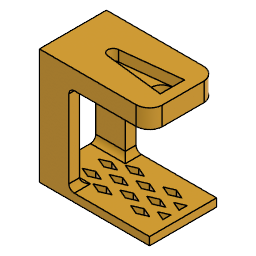
femur (Autodesk Fusion 360 design; units mm, degrees)
part number: 2026-05-23-05-17-23-124
Autodesk Fusion 360 part; units mm, degrees
note: some values were not read from the file. Set by a fixed rule: which face or edge a step refers to.
sketch "Sketch1" plane through (0, 0, 0) normal (0, 1, 0) x (1, 0, 0)
  line L0 (0, 0) -> (0, -33)
  line L1 (0, -33) -> (41, -33)
  line L2 (41, -33) -> (41, 0)
  line L3 (41, 0) -> (0, 0)
  dimension "d1" = 33
  dimension "d2" = 41
  constraint coincident L0.start L3.end
  constraint vertical L0
  constraint perpendicular L0 L1
  constraint perpendicular L1 L2
  constraint perpendicular L0 L3
  measures "d1" distance of L0.start L0.end
  measures "d2" distance of L0.end L1.end
extrude "Extrude1" add sketch "Sketch1" along normal blind 3 contours L0 L1 L2 L3 picked at (13.666667, -22)
sketch "Sketch2" plane through (0, 3, 0) normal (0, 1, 0) x (-1, 0, 0)
  line L0 (-41, 0) -> (0, 0)
  line L1 (0, 0) -> (0, 33)
  line L2 (0, 33) -> (-41, 33)
  line L3 (-41, 33) -> (-41, 0)
  line L4 (-41, 33) -> (-41, 30)
  line L5 (-41, 30) -> (0, 30)
  line L6 (0, 30) -> (0, 33)
  line L7 (0, 33) -> (-41, 33)
  line L8 (-41, 0) -> (-41, 3)
  line L9 (-41, 3) -> (0, 3)
  line L10 (0, 3) -> (0, 0)
  line L11 (0, 0) -> (-41, 0)
  constraint coincident L2.end L3.start
  constraint coincident L3 L4.end
  constraint coincident L1 L5.end
  constraint perpendicular L1 L5
  constraint coincident L1.end L2.start
  constraint coincident L0.start L3.end
  constraint coincident L3 L8.end
  constraint coincident L1 L9.end
  constraint perpendicular L1 L9
  constraint coincident L0.end L1.start
extrude "Extrude2" add sketch "Sketch2" along normal blind 15 contours L0 L1 L3 L8 L9 L10 L11 | L1 L2 L3 L4 L5 L6 L7 picked at (-27.333333, 2) picked at (-27.333333, 32)
sketch "Sketch3" plane through (0, 18, 0) normal (0, 1, 0) x (-1, 0, 0)
  line L0 (0, 33) -> (-41, 33)
  line L1 (-41, 33) -> (-41, 30)
  line L2 (-41, 30) -> (0, 30)
  line L3 (0, 30) -> (0, 33)
  line L4 (-41, 33) -> (-41, 30)
  line L5 (-41, 30) -> (0, 30)
  line L6 (0, 30) -> (0, 33)
  line L7 (0, 33) -> (-41, 33)
  line L8 (-41, 30) -> (-38.000001, 30)
  line L9 (-38.000001, 30) -> (-38.000001, 0)
  line L10 (-38.000001, 0) -> (-41, 0)
  line L11 (-41, 0) -> (-41, 30)
  line L12 (0, 0) -> (-3, 0)
  line L13 (-3, 0) -> (-3, 30)
  line L14 (0, 30) -> (0, 0)
  line L15 (-41.000001, 3) -> (0, 3)
  line L16 (0, 0) -> (-38.000001, 0)
  line L17 (-38.000001, 30) -> (-31.000001, 30)
  line L18 (-31.000001, 30) -> (-24.000001, 30)
  line L19 (-24.000001, 30) -> (-17.000001, 30)
  line L20 (-17.000001, 30) -> (-10.000001, 30)
  line L21 (-10.000001, 30) -> (-3, 30)
  line L22 (-38.000001, 30) -> (-38.000001, 24.6)
  line L23 (-38.000001, 24.6) -> (-38.000001, 19.2)
  line L24 (-38.000001, 19.2) -> (-38.000001, 13.8)
  line L25 (-38.000001, 13.8) -> (-38.000001, 8.4)
  line L26 (-38.000001, 3) -> (-31.000001, 3)
  line L27 (-31.000001, 3) -> (-24.000001, 3)
  line L28 (-24.000001, 3) -> (-17.000001, 3)
  line L29 (-17.000001, 3) -> (-10, 3)
  line L30 (-3, 3) -> (-3, 8.4)
  line L31 (-3, 8.4) -> (-3, 13.8)
  line L32 (-3, 13.8) -> (-3, 19.2)
  line L33 (-3, 19.2) -> (-3, 24.6)
  line L34 (-38.000001, 30) -> (-3, 3)
  line L35 (-38.000001, 24.6) -> (-10, 3)
  line L36 (-38.000001, 19.2) -> (-17.000001, 3)
  line L37 (-38.000001, 13.8) -> (-24, 3)
  line L38 (-38.000001, 8.4) -> (-31.000001, 3)
  line L39 (-31.000001, 30) -> (-3, 8.4)
  line L40 (-24.000001, 30) -> (-3, 13.8)
  line L41 (-17.000001, 30) -> (-3, 19.2)
  line L42 (-10.000001, 30) -> (-3, 24.6)
  line L43 (-3, 30) -> (-38.000001, 3)
  line L44 (-3, 24.6) -> (-31.000001, 3)
  line L45 (-3, 19.2) -> (-24.000001, 3)
  line L46 (-3, 13.8) -> (-17.000001, 3)
  line L47 (-3, 8.4) -> (-10, 3)
  line L48 (-10.000001, 30) -> (-38.000001, 8.4)
  line L49 (-17.000001, 30) -> (-38.000001, 13.8)
  line L50 (-24.000001, 30) -> (-38.000001, 19.2)
  line L51 (-31.000001, 30) -> (-38.000001, 24.6)
  dimension "d7" = 7
  dimension "d8" = 7
  dimension "d9" = 7
  dimension "d10" = 7
  dimension "d11" = 5.4
  dimension "d12" = 5.4
  dimension "d13" = 5.4
  dimension "d14" = 5.4
  dimension "d15" = 7
  dimension "d16" = 7
  dimension "d17" = 7
  dimension "d18" = 7
  dimension "d19" = 5.4
  dimension "d20" = 5.4
  dimension "d21" = 5.4
  dimension "d22" = 5.4
  constraint coincident L0.end L1.start
  constraint coincident L1.end L2.start
  constraint coincident L2.end L3.start
  constraint coincident L0.start L3.end
  constraint perpendicular L8 L9
  constraint perpendicular L9 L10
  constraint perpendicular L5 L11
  constraint coincident L12.start L14.end
  constraint perpendicular L9 L12
  constraint coincident L5 L13.end
  constraint perpendicular L5 L13
  constraint coincident L14 L15.end
  constraint perpendicular L14 L15
  constraint perpendicular L9 L16
  constraint perpendicular L13 L17
  constraint perpendicular L13 L18
  constraint perpendicular L13 L19
  constraint perpendicular L13 L20
  constraint perpendicular L21 L22
  constraint parallel L9 L23
  constraint parallel L9 L24
  constraint parallel L9 L25
  constraint perpendicular L9 L26
  constraint perpendicular L9 L27
  constraint parallel L15 L28
  constraint coincident L15 L29.end
  constraint coincident L13 L30.start
  constraint coincident L15 L30.start
  constraint perpendicular L15 L30
  constraint parallel L13 L31
  constraint parallel L13 L32
  constraint parallel L13 L33
  constraint parallel L36 L37
  constraint parallel L39 L40
  measures "d19" distance of L30.start L30.end
  measures "d20" distance of L30.end L31.end
  measures "d21" distance of L31.end L32.end
  measures "d22" distance of L32.end L33.end
extrude "Extrude3" add sketch "Sketch3" along normal blind 3 contours L0 L1 L2 L3 L4 L5 L6 L7 L8 L17 L18 L19 L20 L21 | L2 L5 L13 L14 L15 L30 L31 L32 L33 | L2 L5 L8 L9 L11 L15 L22 L23 L24 L25 | L2 L5 L21 L42 L43 | L13 L42 L43 | L12 L13 L14 L15 L16 | L9 L22 L34 L51 | L2 L5 L17 L34 L51 | L9 L10 L11 L15 | L41 L42 L43 L48 | L13 L33 L41 L44 | L13 L30 L34 L47 | L9 L13 L15 L16 L26 L27 L28 L29 | L34 L39 L50 L51 | L9 L23 L35 L50 | L9 L38 L43 | L2 L5 L19 L40 L49 | L40 L41 L48 L49 | L40 L41 L43 L48 | L40 L41 L44 L45 | L13 L32 L40 L45 | L40 L41 L43 L44 | L13 L31 L39 L46 | L34 L39 L46 L47 | L15 L29 L35 L46 | L34 L35 L46 L47 | L39 L40 L49 L50 | L34 L39 L49 L50 | L9 L24 L36 L49 | L35 L36 L49 L50 | L34 L35 L49 L50 | L37 L38 L43 L48 | L9 L25 L37 L48 | L15 L27 L37 L44 | L37 L38 L43 L44 | L39 L40 L43 L48 | L39 L40 L44 L45 | L34 L39 L45 L46 | L35 L36 L45 L46 | L34 L39 L48 L49 | L35 L36 L48 L49 | L36 L37 L43 L48 | L36 L37 L44 L45 | L34 L39 L43 L48 | L34 L39 L44 L45 | L34 L39 L43 L44 | L35 L36 L44 L45 | L34 L35 L44 L45 | L35 L36 L43 L48 | L34 L35 L43 L48 | L35 L36 L43 L44 picked at (-24, 32) picked at (-1, 17.4) picked at (-40, 15.6) picked at (-6.5, 29.1) picked at (-4.166667, 27.3) picked at (-2, 2) picked at (-36.833334, 27.3) picked at (-34.500001, 29.1) picked at (-40, 2) picked at (-8.833334, 27.3) picked at (-4.166667, 21.9) picked at (-4.166667, 5.7) picked at (-19.333334, 1) picked at (-29.833334, 27.3) picked at (-36.833334, 21.9) picked at (-36.833334, 5.7) picked at (-20.500001, 29.1) picked at (-18.166667, 27.3) picked at (-14.666667, 24.6) picked at (-5.333333, 19.2) picked at (-4.166667, 16.5) picked at (-8.833333, 21.9) picked at (-4.166667, 11.1) picked at (-7.666667, 8.4) picked at (-13.5, 3.9) picked at (-11.166667, 5.7) picked at (-25.166667, 27.3) picked at (-26.333334, 24.6) picked at (-36.833334, 16.5) picked at (-33.333334, 19.2) picked at (-29.833334, 21.9) picked at (-33.333334, 8.4) picked at (-36.833334, 11.1) picked at (-27.500001, 3.9) picked at (-29.833334, 5.7) picked at (-18.166667, 21.9) picked at (-8.833333, 16.5) picked at (-8.833333, 11.1) picked at (-15.833334, 5.7) picked at (-25.166667, 21.9) picked at (-29.833334, 16.5) picked at (-29.833334, 11.1) picked at (-22.833334, 5.7) picked at (-19.333334, 19.2) picked at (-12.333333, 13.8) picked at (-15.833334, 16.5) picked at (-19.333334, 8.4) picked at (-15.833334, 11.1) picked at (-26.333334, 13.8) picked at (-22.833334, 16.5) picked at (-22.833334, 11.1)
sketch "Sketch4" plane through (0, 0, 0) normal (0, -1, 0) x (1, 0, 0)
  line L0 (0, 0) -> (41, 0)
  line L1 (41, 0) -> (41, 33)
  line L2 (41, 33) -> (0, 33)
  line L3 (0, 33) -> (0, 0)
  line L4 (0, 33) -> (0, 30)
  line L5 (0, 30) -> (41, 30)
  line L6 (41, 30) -> (41, 33)
  line L7 (0, 33) -> (41, 33)
  line L8 (0, 0) -> (0, 3)
  line L9 (0, 3) -> (41, 3)
  line L10 (41, 3) -> (41, 0)
  line L11 (41, 0) -> (0, 0)
  line L12 (0, 33) -> (3, 33)
  line L13 (3, 33) -> (3, 3)
  line L14 (41, 33) -> (38.000001, 33)
  line L15 (38.000001, 33) -> (38.000001, 3)
  line L16 (3, 30) -> (3, 24.6)
  line L17 (3, 24.6) -> (3, 19.2)
  line L18 (3, 19.2) -> (3, 13.8)
  line L19 (3, 13.8) -> (3, 8.4)
  line L20 (3, 3) -> (10, 3)
  line L21 (10, 3) -> (17, 3)
  line L22 (17, 3) -> (24, 3)
  line L23 (24, 3) -> (31, 3)
  line L24 (38.000001, 3) -> (38.000001, 8.4)
  line L25 (38.000001, 8.4) -> (38.000001, 13.8)
  line L26 (38.000001, 13.8) -> (38.000001, 19.2)
  line L27 (38.000001, 19.2) -> (38.000001, 24.6)
  line L28 (38.000001, 30) -> (31.000001, 30)
  line L29 (31.000001, 30) -> (24.000001, 30)
  line L30 (24.000001, 30) -> (17.000001, 30)
  line L31 (17.000001, 30) -> (10.000001, 30)
  line L32 (3, 30) -> (38.000001, 3)
  line L33 (3, 24.6) -> (31, 3)
  line L34 (3, 19.2) -> (24, 3)
  line L35 (3, 13.8) -> (17, 3)
  line L36 (3, 8.4) -> (10, 3)
  line L37 (10.000001, 30) -> (38.000001, 8.4)
  line L38 (17.000001, 30) -> (38.000001, 13.8)
  line L39 (24.000001, 30) -> (38.000001, 19.2)
  line L40 (31.000001, 30) -> (38.000001, 24.6)
  line L41 (38.000001, 30) -> (3, 3)
  line L42 (38.000001, 24.6) -> (10, 3)
  line L43 (38.000001, 19.2) -> (17, 3)
  line L44 (38.000001, 13.8) -> (24, 3)
  line L45 (38.000001, 8.4) -> (31, 3)
  line L46 (31.000001, 30) -> (3, 8.4)
  line L47 (24.000001, 30) -> (3, 13.8)
  line L48 (17.000001, 30) -> (3, 19.2)
  line L49 (10.000001, 30) -> (3, 24.6)
  dimension "d25" = 5.4
  dimension "d26" = 5.4
  dimension "d27" = 5.4
  dimension "d28" = 5.4
  dimension "d29" = 7
  dimension "d30" = 7
  dimension "d31" = 7
  dimension "d32" = 7
  dimension "d33" = 5.4
  dimension "d34" = 5.4
  dimension "d35" = 5.4
  dimension "d36" = 5.4
  dimension "d37" = 7
  dimension "d38" = 7
  dimension "d39" = 7
  dimension "d40" = 7
  constraint coincident L2.end L3.start
  constraint coincident L3 L4.end
  constraint coincident L1 L5.end
  constraint perpendicular L1 L5
  constraint coincident L1.end L2.start
  constraint coincident L0.start L3.end
  constraint coincident L3 L8.end
  constraint perpendicular L3 L9
  constraint coincident L0.end L1.start
  constraint perpendicular L9 L10
  constraint coincident L7 L12.end
  constraint coincident L9 L13.end
  constraint perpendicular L9 L13
  constraint perpendicular L9 L15
  constraint coincident L13 L16.start
  constraint coincident L5 L16.start
  constraint perpendicular L5 L16
  constraint parallel L13 L17
  constraint parallel L13 L18
  constraint parallel L13 L19
  constraint perpendicular L13 L20
  constraint perpendicular L13 L21
  constraint parallel L9 L22
  constraint parallel L9 L23
  constraint perpendicular L9 L24
  constraint parallel L15 L26
  constraint parallel L15 L27
  constraint perpendicular L15 L28
  constraint perpendicular L15 L29
  constraint parallel L5 L30
  constraint parallel L5 L31
  measures "d25" distance of L16.start L16.end
  measures "d26" distance of L16.end L17.end
  measures "d27" distance of L17.end L18.end
  measures "d28" distance of L18.end L19.end
  measures "d29" distance of L13.end L20.end
  measures "d30" distance of L20.end L21.end
  measures "d31" distance of L21.end L22.end
  measures "d32" distance of L22.end L23.end
extrude "Extrude4" cut sketch "Sketch4" against normal blind 10 contours L9 L20 L36 L41 | L9 L32 L45 | L5 L31 L37 L48 | L32 L33 L48 L49 | L9 L22 L34 L43 | L34 L35 L41 L42 | L34 L35 L46 L47 | L5 L29 L39 L46 | L39 L40 L41 L42 | L32 L33 L43 L44 | L37 L38 L43 L44 | L37 L38 L46 L47 | L32 L33 L46 L47 | L32 L33 L41 L42 | L37 L38 L41 L42 picked at (6.5, 3.9) picked at (34.5, 3.9) picked at (13.500001, 29.1) picked at (5.333333, 24.6) picked at (20.5, 3.9) picked at (14.666667, 8.4) picked at (7.666667, 13.8) picked at (27.500001, 29.1) picked at (33.333334, 24.6) picked at (28.666667, 8.4) picked at (35.666667, 13.8) picked at (19.333334, 24.6) picked at (14.666667, 19.2) picked at (21.666667, 13.8) picked at (28.666667, 19.2)
sketch "Sketch5" plane through (0, 0, 33) normal (0, 0, 1) x (-1, 0, 0)
  line L0 (0, 0) -> (-41, 0)
  line L1 (-41, 0) -> (-41, -21)
  line L2 (-41, -21) -> (0, -21)
  line L3 (0, -21) -> (0, 0)
  line L4 (-41, -21) -> (-41, -10.5)
  line L5 (-41, -10.5) -> (-36.5, -10.5)
  circle A0 centre (-36.5, -10.5) radius 1.25
  dimension "d43" = 4.5
  dimension "d44" = 2.5
  constraint coincident L1.end L2.start
  constraint midpoint L1 L4.end
  constraint perpendicular L1 L5
  constraint coincident L5.end A0.centre
  measures "d43" distance of L4.end L5.end
  measures "d44" diameter of A0
extrude "Extrude5" add sketch "Sketch5" along normal blind 4 contours L0 L1 L2 L3 L4 picked at (-11.75, -10.5)
extrude "Extrude6" cut 1 faces at (36.347775, 11.012066, 33) along direction (0, 0, -1) blind 1.5
extrude "Extrude7" add 1 faces at (36.347775, 11.012066, 31.5) along direction (0, 0, 1) blind 5.5
sketch "Sketch6" plane through (0, 0, 30) normal (0, 0, -1) x (1, 0, 0)
  line L0 (10.000001, -3) -> (0, -3)
  line L1 (0, -3) -> (0, -18)
  line L2 (0, -18) -> (10.000001, -18)
  line L3 (10.000001, -18) -> (10.000001, -21)
  line L4 (10.000001, -21) -> (17.000001, -21)
  line L5 (17.000001, -21) -> (17.000001, -18)
  line L6 (17.000001, -18) -> (24.000001, -18)
  line L7 (24.000001, -18) -> (24.000001, -21)
  line L8 (24.000001, -21) -> (31.000001, -21)
  line L9 (31.000001, -21) -> (31.000001, -18)
  line L10 (31.000001, -18) -> (41, -18)
  line L11 (41, -18) -> (41, -3)
  line L12 (41, -3) -> (31.000001, -3)
  line L13 (31.000001, -3) -> (31.000001, 0)
  line L14 (31.000001, 0) -> (24.000001, 0)
  line L15 (24.000001, 0) -> (24.000001, -3)
  line L16 (24.000001, -3) -> (17.000001, -3)
  line L17 (17.000001, -3) -> (17.000001, 0)
  line L18 (17.000001, 0) -> (10.000001, 0)
  line L19 (10.000001, 0) -> (10.000001, -3)
  line L20 (0, -21) -> (0, -10.5)
  line L21 (0, -10.5) -> (4.5, -10.5)
  circle A0 centre (4.5, -10.5) radius 1.25
  dimension "d51" = 4.5
  dimension "d52" = 2.5
  constraint midpoint L1 L20.end
  constraint perpendicular L2 L20
  constraint perpendicular L20 L21
  constraint coincident L21.end A0.centre
  measures "d51" distance of L20.end L21.end
  measures "d52" diameter of A0
extrude "Extrude8" cut sketch "Sketch6" against normal blind 5.5 contours A0 picked at (4.839612, -10.203182)
sketch "Sketch7" plane through (0, 0, 37) normal (0, 0, 1) x (-1, 0, 0)
  line L0 (0, -21) -> (0, 0)
  line L1 (0, 0) -> (-41, 0)
  line L2 (-41, 0) -> (-41, -21)
  line L3 (-41, -21) -> (0, -21)
  line L4 (-41, -10.5) -> (-37, -10.5)
  line L5 (-37, -10.5) -> (-37, -6)
  line L6 (-37, -6) -> (-37, -15)
  line L7 (-37, -10.5) -> (-15, -10.5)
  line L8 (-15, -10.5) -> (-15, -12.5)
  line L9 (-15, -12.5) -> (-15, -8.5)
  line L10 (-15, -8.5) -> (-37, -6)
  line L11 (-15, -12.5) -> (-37, -15)
  circle A0 centre (-15, -10.5) radius 2
  dimension "d55" = 4
  dimension "d56" = 4.5
  dimension "d57" = 9
  dimension "d58" = 22
  dimension "d59" = 2
  dimension "d60" = 4
  dimension "d61" = 4
  constraint midpoint L2 L4.start
  constraint perpendicular L2 L4
  constraint perpendicular L4 L5
  constraint parallel L5 L6
  constraint perpendicular L5 L7
  constraint perpendicular L7 L8
  constraint perpendicular L7 L9
  constraint coincident L7.end L8.start
  measures "d55" distance of L4.start L4.end
  measures "d56" distance of L4.end L5.end
  measures "d57" distance of L5.end L6.end
  measures "d58" distance of L4.end L7.end
  measures "d59" distance of L7.end L8.end
  measures "d60" distance of L8.end L9.end
  measures "d61" diameter of A0
extrude "Extrude9" cut sketch "Sketch7" against normal blind 4 contours L6 L7 L11 A0 | L5 L6 L7 L10 A0 | L7 L9 A0 | L7 L8 L9 A0 | L8 L9 A0 picked at (-30.326548, -12.094877) picked at (-30.326548, -8.905123) picked at (-15.797001, -9.435331) picked at (-16.326548, -10.594877) picked at (-13.673452, -10.594877)
sketch "Sketch8" plane through (0, 0, 33) normal (0, 0, 1) x (-1, 0, 0)
  arc A0 (-15, -12.5) -> (-15, -8.5) centre (-15, -10.5) ccw
  line L0 (-15, -8.5) -> (-37, -6)
  line L1 (-37, -6) -> (-37, -15)
  line L2 (-37, -15) -> (-15, -12.5)
  line L3 (-37, -10.5) -> (-33, -10.5)
  circle A1 centre (-33, -10.5) radius 3.75
  dimension "d64" = 4
  dimension "d65" = 7.5
  constraint midpoint L1 L3.start
  constraint perpendicular L1 L3
  constraint coincident L3.end A1.centre
  measures "d64" distance of L3.start L3.end
  measures "d65" diameter of A1
extrude "Extrude10" cut sketch "Sketch8" against normal blind 10 contours A1 picked at (-32.220638, -9.522711)
sketch "Sketch9" plane through (0, 0, 0) normal (0, 0, -1) x (1, 0, 0)
  line L0 (41, 0) -> (0, 0)
  line L1 (0, 0) -> (0, -21)
  line L2 (0, -21) -> (41, -21)
  line L3 (41, -21) -> (41, 0)
  line L4 (0, 0) -> (0, -3)
  line L5 (0, -3) -> (41, -3)
  line L6 (0, -21) -> (0, -18)
  line L7 (0, -18) -> (41, -18)
  line L8 (0, -3) -> (3, -3)
  line L9 (3, -3) -> (3, -18)
  line L10 (41, -3) -> (38, -3)
  line L11 (38, -3) -> (38, -18)
  line L12 (3, -3) -> (10, -3)
  line L13 (3, -3) -> (10, -3)
  line L14 (10, -3) -> (17, -3)
  line L15 (17, -3) -> (24, -3)
  line L16 (24, -3) -> (31, -3)
  line L17 (38, -3) -> (38, -6)
  line L18 (38, -6) -> (38, -9)
  line L19 (38, -9) -> (38, -12)
  line L20 (38, -12) -> (38, -15)
  line L21 (38, -18) -> (31, -18)
  line L22 (31, -18) -> (24, -18)
  line L23 (24, -18) -> (17, -18)
  line L24 (17, -18) -> (10, -18)
  line L25 (3, -18) -> (3, -15)
  line L26 (3, -15) -> (3, -12)
  line L27 (3, -12) -> (3, -9)
  line L28 (3, -9) -> (3, -6)
  line L29 (3, -3) -> (38, -18)
  line L30 (3, -6) -> (31, -18)
  line L31 (3, -9) -> (24, -18)
  line L32 (3, -12) -> (17, -18)
  line L33 (3, -15) -> (10, -18)
  line L34 (10, -3) -> (38, -15)
  line L35 (17, -3) -> (38, -12)
  line L36 (24, -3) -> (38, -9)
  line L37 (31, -3) -> (38, -6)
  line L38 (38, -3) -> (3, -18)
  line L39 (38, -6) -> (10, -18)
  line L40 (38, -9) -> (17, -18)
  line L41 (38, -12) -> (24, -18)
  line L42 (38, -15) -> (31, -18)
  line L43 (31, -3) -> (3, -15)
  line L44 (24, -3) -> (3, -12)
  line L45 (17, -3) -> (3, -9)
  line L46 (10, -3) -> (3, -6)
  dimension "d68" = 3
  dimension "d69" = 3
  dimension "d70" = 7
  dimension "d71" = 7
  dimension "d72" = 7
  dimension "d73" = 7
  dimension "d74" = 3
  dimension "d75" = 3
  dimension "d76" = 3
  dimension "d77" = 3
  dimension "d78" = 7
  dimension "d79" = 7
  dimension "d80" = 7
  dimension "d81" = 7
  dimension "d82" = 3
  dimension "d83" = 3
  dimension "d84" = 3
  dimension "d85" = 3
  constraint coincident L0.end L1.start
  constraint perpendicular L0 L4
  constraint coincident L3 L5.end
  constraint perpendicular L3 L5
  constraint coincident L1.end L2.start
  constraint coincident L1 L6.end
  constraint coincident L3 L7.end
  constraint perpendicular L3 L7
  constraint coincident L5 L8.end
  constraint coincident L7 L9.end
  constraint perpendicular L7 L9
  constraint perpendicular L3 L10
  constraint coincident L7 L11.end
  constraint perpendicular L7 L11
  constraint coincident L5 L12.end
  constraint perpendicular L9 L13
  constraint parallel L5 L14
  constraint parallel L5 L15
  constraint parallel L5 L16
  constraint perpendicular L10 L17
  constraint perpendicular L10 L18
  constraint parallel L11 L19
  constraint parallel L11 L20
  constraint perpendicular L11 L21
  constraint perpendicular L11 L22
  constraint parallel L7 L23
  constraint parallel L7 L24
  constraint perpendicular L7 L25
  constraint perpendicular L7 L26
  constraint parallel L9 L27
  constraint parallel L9 L28
  measures "d68" distance of L0.end L4.end
  measures "d69" distance of L5.end L10.end
  measures "d70" distance of L8.end L12.end
  measures "d71" distance of L12.end L14.end
  measures "d72" distance of L14.end L15.end
  measures "d73" distance of L15.end L16.end
  measures "d74" distance of L10.end L17.end
  measures "d75" distance of L17.end L18.end
  measures "d76" distance of L18.end L19.end
  measures "d77" distance of L19.end L20.end
  measures "d78" distance of L11.end L21.end
  measures "d79" distance of L21.end L22.end
  measures "d80" distance of L22.end L23.end
  measures "d81" distance of L23.end L24.end
  measures "d82" distance of L9.end L25.end
  measures "d83" distance of L25.end L26.end
  measures "d84" distance of L26.end L27.end
  measures "d85" distance of L27.end L28.end
extrude "Extrude11" cut sketch "Sketch9" against normal blind 10 contours L9 L29 L46 | L36 L37 L38 L43 | L11 L18 L36 L39 | L9 L25 L33 L38 | L29 L30 L41 L42 | L11 L20 L34 L41 | L34 L35 L44 L45 | L9 L27 L31 L44 | L29 L30 L44 L45 | L34 L35 L38 L43 | L34 L35 L39 L40 | L31 L32 L39 L40 | L31 L32 L38 L43 | L29 L30 L39 L40 | L29 L30 L38 L43 picked at (4.166667, -4.5) picked at (29.833333, -4.5) picked at (36.833333, -7.5) picked at (4.166667, -16.5) picked at (29.833333, -16.5) picked at (36.833333, -13.5) picked at (18.166667, -4.5) picked at (4.166667, -10.5) picked at (8.833333, -7.5) picked at (25.166667, -7.5) picked at (29.833333, -10.5) picked at (15.833333, -16.5) picked at (11.166667, -13.5) picked at (22.833333, -13.5) picked at (15.833333, -10.5)
extrude "Extrude12" cut 1 faces at (19.333333, 20, 0) along direction (0, 0, 1) blind 1
extrude "Extrude13" add 1 faces at (19.333333, 20, 1) along direction (0, 0, -1) blind 9
extrude "Extrude14" cut 1 faces at (20.5, 10.5, 3) along direction (0, 0, -1) blind 9
sketch "Sketch10" plane through (0, 21, 0) normal (0, 1, 0) x (-1, 0, 0)
  line L0 (0, -8) -> (0, 37)
  line L1 (0, 37) -> (-41, 37)
  line L2 (-41, 37) -> (-41, -8)
  line L3 (-41, -8) -> (0, -8)
  line L4 (-13.500001, 27.3) -> (-17.000001, 30)
  line L5 (-17.000001, 30) -> (-10.000001, 30)
  line L6 (-10.000001, 30) -> (-13.500001, 27.3)
  line L7 (-27.500001, 27.3) -> (-31.000001, 30)
  line L8 (-31.000001, 30) -> (-24.000001, 30)
  line L9 (-24.000001, 30) -> (-27.500001, 27.3)
  line L10 (-34.500001, 21.9) -> (-38.000001, 24.6)
  line L11 (-38.000001, 24.6) -> (-34.500001, 27.3)
  line L12 (-34.500001, 27.3) -> (-31.000001, 24.6)
  line L13 (-31.000001, 24.6) -> (-34.500001, 21.9)
  line L14 (-13.5, 5.7) -> (-17, 8.4)
  line L15 (-17, 8.4) -> (-13.5, 11.1)
  line L16 (-13.5, 11.1) -> (-10, 8.4)
  line L17 (-10, 8.4) -> (-13.5, 5.7)
  line L18 (-34.500001, 11.1) -> (-38.000001, 13.8)
  line L19 (-38.000001, 13.8) -> (-34.500001, 16.5)
  line L20 (-34.500001, 16.5) -> (-31.000001, 13.8)
  line L21 (-31.000001, 13.8) -> (-34.500001, 11.1)
  line L22 (-10, 24.6) -> (-6.5, 27.3)
  line L23 (-6.5, 27.3) -> (-3, 24.6)
  line L24 (-3, 24.6) -> (-6.5, 21.9)
  line L25 (-6.5, 21.9) -> (-10, 24.6)
  line L26 (-13.5, 16.5) -> (-17, 19.2)
  line L27 (-17, 19.2) -> (-13.5, 21.9)
  line L28 (-13.5, 21.9) -> (-10, 19.2)
  line L29 (-10, 19.2) -> (-13.5, 16.5)
  line L30 (-27.500001, 16.5) -> (-31.000001, 19.2)
  line L31 (-31.000001, 19.2) -> (-27.500001, 21.9)
  line L32 (-27.500001, 21.9) -> (-24.000001, 19.2)
  line L33 (-24.000001, 19.2) -> (-27.500001, 16.5)
  line L34 (-31.000001, 3) -> (-31.000001, -6)
  line L35 (-31.000001, -6) -> (-38.000001, -6)
  line L36 (-38.000001, -6) -> (-38.000001, 3)
  line L37 (-38.000001, 3) -> (-34.5, 5.7)
  line L38 (-34.5, 5.7) -> (-31.000001, 3)
  line L39 (-20.500001, 21.9) -> (-24.000001, 24.6)
  line L40 (-24.000001, 24.6) -> (-20.500001, 27.3)
  line L41 (-20.500001, 27.3) -> (-17.000001, 24.6)
  line L42 (-17.000001, 24.6) -> (-20.500001, 21.9)
  line L43 (-27.5, 5.7) -> (-31, 8.4)
  line L44 (-31, 8.4) -> (-27.5, 11.1)
  line L45 (-27.5, 11.1) -> (-24, 8.4)
  line L46 (-24, 8.4) -> (-27.5, 5.7)
  line L47 (-20.5, 11.1) -> (-24, 13.8)
  line L48 (-24, 13.8) -> (-20.5, 16.5)
  line L49 (-20.5, 16.5) -> (-17, 13.8)
  line L50 (-17, 13.8) -> (-20.5, 11.1)
  line L51 (-10, 13.8) -> (-6.5, 16.5)
  line L52 (-6.5, 16.5) -> (-3, 13.8)
  line L53 (-3, 13.8) -> (-6.5, 11.1)
  line L54 (-6.5, 11.1) -> (-10, 13.8)
  line L55 (-10, -6) -> (-10, 3)
  line L56 (-10, 3) -> (-6.5, 5.7)
  line L57 (-6.5, 5.7) -> (-3, 3)
  line L58 (-3, 3) -> (-3, -6)
  line L59 (-3, -6) -> (-10, -6)
  line L60 (-24.000001, -6) -> (-24.000001, 3)
  line L61 (-24.000001, 3) -> (-20.5, 5.7)
  line L62 (-20.5, 5.7) -> (-17.000001, 3)
  line L63 (-17.000001, 3) -> (-17.000001, -6)
  line L64 (-17.000001, -6) -> (-24.000001, -6)
  line L65 (-38.000001, -6) -> (-38.000001, -4)
  line L66 (-38.000001, -4) -> (-31.000001, -4)
  line L67 (-41.000001, -4) -> (-38.000001, -4)
  line L68 (-31.000001, -4) -> (0, -4)
  constraint perpendicular L34 L66
  constraint perpendicular L36 L67
  constraint coincident L0 L68.end
  constraint perpendicular L0 L68
extrude "Extrude15" add sketch "Sketch10" against normal blind 3 contours L55 L58 L59 L68 | L34 L35 L36 L65 L66 | L60 L63 L64 L68 picked at (-7.666667, -4.666667) picked at (-35.666667, -4.666667) picked at (-21.666667, -4.666667)
sketch "Sketch11" plane through (0, 0, 0) normal (0, -1, 0) x (1, 0, 0)
  line L0 (24, 3) -> (24, -6)
  line L1 (24, -6) -> (17, -6)
  line L2 (17, -6) -> (17, 3)
  line L3 (17, 3) -> (20.5, 5.7)
  line L4 (20.5, 5.7) -> (24, 3)
  line L5 (34.500001, 21.9) -> (31, 24.6)
  line L6 (31, 24.6) -> (34.5, 27.3)
  line L7 (34.5, 27.3) -> (38.000001, 24.6)
  line L8 (38.000001, 24.6) -> (34.500001, 21.9)
  line L9 (31.000001, 30) -> (27.5, 27.3)
  line L10 (27.5, 27.3) -> (24.000001, 30)
  line L11 (24.000001, 30) -> (31.000001, 30)
  line L12 (17, 19.2) -> (13.5, 16.5)
  line L13 (13.5, 16.5) -> (10, 19.2)
  line L14 (10, 19.2) -> (13.5, 21.9)
  line L15 (13.5, 21.9) -> (17, 19.2)
  line L16 (10, 24.6) -> (6.5, 21.9)
  line L17 (6.5, 21.9) -> (3, 24.6)
  line L18 (3, 24.6) -> (6.5, 27.3)
  line L19 (6.5, 27.3) -> (10, 24.6)
  line L20 (38.000001, 3) -> (38.000001, -6)
  line L21 (38.000001, -6) -> (31, -6)
  line L22 (31, -6) -> (31, 3)
  line L23 (31, 3) -> (34.5, 5.7)
  line L24 (34.5, 5.7) -> (38.000001, 3)
  line L25 (31.000001, 19.2) -> (27.500001, 16.5)
  line L26 (27.500001, 16.5) -> (24, 19.2)
  line L27 (24, 19.2) -> (27.5, 21.9)
  line L28 (27.5, 21.9) -> (31.000001, 19.2)
  line L29 (34.500001, 11.1) -> (31.000001, 13.8)
  line L30 (31.000001, 13.8) -> (34.500001, 16.5)
  line L31 (34.500001, 16.5) -> (38.000001, 13.8)
  line L32 (38.000001, 13.8) -> (34.500001, 11.1)
  line L33 (17, 8.4) -> (13.5, 5.7)
  line L34 (13.5, 5.7) -> (10, 8.4)
  line L35 (10, 8.4) -> (13.5, 11.1)
  line L36 (13.5, 11.1) -> (17, 8.4)
  line L37 (10, 13.8) -> (6.5, 11.1)
  line L38 (6.5, 11.1) -> (3, 13.8)
  line L39 (3, 13.8) -> (6.5, 16.5)
  line L40 (6.5, 16.5) -> (10, 13.8)
  line L41 (24, 13.8) -> (20.5, 11.1)
  line L42 (20.5, 11.1) -> (17, 13.8)
  line L43 (17, 13.8) -> (20.5, 16.5)
  line L44 (20.5, 16.5) -> (24, 13.8)
  line L45 (24, 24.6) -> (20.5, 21.9)
  line L46 (20.5, 21.9) -> (17, 24.6)
  line L47 (17, 24.6) -> (20.5, 27.3)
  line L48 (20.5, 27.3) -> (24, 24.6)
  line L49 (31, 8.4) -> (27.5, 5.7)
  line L50 (27.5, 5.7) -> (24, 8.4)
  line L51 (24, 8.4) -> (27.5, 11.1)
  line L52 (27.5, 11.1) -> (31, 8.4)
  line L53 (17.000001, 30) -> (13.5, 27.3)
  line L54 (13.5, 27.3) -> (10.000001, 30)
  line L55 (10.000001, 30) -> (17.000001, 30)
  line L56 (10, 3) -> (10, -6)
  line L57 (10, -6) -> (3, -6)
  line L58 (3, -6) -> (3, 3)
  line L59 (3, 3) -> (6.5, 5.7)
  line L60 (6.5, 5.7) -> (10, 3)
  line L61 (41, -8) -> (41, 37)
  line L62 (41, 37) -> (0, 37)
  line L63 (0, 37) -> (0, -8)
  line L64 (0, -8) -> (41, -8)
  line L65 (3, -6) -> (3, -4)
  line L66 (0, -4) -> (3, -4)
  line L67 (3, -4) -> (41, -4)
  constraint coincident L57.end L58.start
  constraint coincident L58 L65.end
  constraint coincident L63 L66.start
  constraint perpendicular L58 L66
  constraint coincident L61 L67.end
  constraint perpendicular L61 L67
extrude "Extrude16" add sketch "Sketch11" against normal blind 3 contours L0 L1 L2 L67 | L20 L21 L22 L67 | L56 L57 L58 L65 L67 picked at (19.333333, -4.666667) picked at (33.333334, -4.666667) picked at (5.333333, -4.666667)
extrude "Extrude17" add 1 faces at (20.5, 13.35, -6) along direction (0, 0, 1) blind 3
extrude "Extrude18" cut 1 faces at (19.333333, 20, -8) along direction (0, 0, 1) blind 3
extrude "Extrude19" add 3 faces at (5.333333, 3, -3.666667) (19.333333, 3, -3.666667) (33.333334, 3, -3.666667) along direction (0, -1, 0) blind 3
extrude "Extrude20" add 3 faces at (33.333334, 18, -3.666667) (19.333334, 18, -3.666667) (5.333333, 18, -3.666667) along direction (0, 1, 0) blind 3
sketch "Sketch12" plane through (0, 0, 0) normal (0, -1, 0) x (1, 0, 0)
  line L0 (0, -5) -> (41, -5)
  line L1 (41, -5) -> (41, 37)
  line L2 (41, 37) -> (0, 37)
  line L3 (0, 37) -> (0, -5)
  line L4 (10, 3) -> (10, -3)
  line L5 (10, -3) -> (3, -3)
  line L6 (3, -3) -> (3, 3)
  line L7 (3, 3) -> (6.5, 5.7)
  line L8 (6.5, 5.7) -> (10, 3)
  line L9 (17.000001, 30) -> (13.5, 27.3)
  line L10 (13.5, 27.3) -> (10.000001, 30)
  line L11 (10.000001, 30) -> (17.000001, 30)
  line L12 (31, 8.4) -> (27.5, 5.7)
  line L13 (27.5, 5.7) -> (24, 8.4)
  line L14 (24, 8.4) -> (27.5, 11.1)
  line L15 (27.5, 11.1) -> (31, 8.4)
  line L16 (24, 24.6) -> (20.5, 21.9)
  line L17 (20.5, 21.9) -> (17, 24.6)
  line L18 (17, 24.6) -> (20.5, 27.3)
  line L19 (20.5, 27.3) -> (24, 24.6)
  line L20 (24, 13.8) -> (20.5, 11.1)
  line L21 (20.5, 11.1) -> (17, 13.8)
  line L22 (17, 13.8) -> (20.5, 16.5)
  line L23 (20.5, 16.5) -> (24, 13.8)
  line L24 (10, 13.8) -> (6.5, 11.1)
  line L25 (6.5, 11.1) -> (3, 13.8)
  line L26 (3, 13.8) -> (6.5, 16.5)
  line L27 (6.5, 16.5) -> (10, 13.8)
  line L28 (17, 8.4) -> (13.5, 5.7)
  line L29 (13.5, 5.7) -> (10, 8.4)
  line L30 (10, 8.4) -> (13.5, 11.1)
  line L31 (13.5, 11.1) -> (17, 8.4)
  line L32 (34.500001, 11.1) -> (31.000001, 13.8)
  line L33 (31.000001, 13.8) -> (34.500001, 16.5)
  line L34 (34.500001, 16.5) -> (38.000001, 13.8)
  line L35 (38.000001, 13.8) -> (34.500001, 11.1)
  line L36 (31.000001, 19.2) -> (27.500001, 16.5)
  line L37 (27.500001, 16.5) -> (24, 19.2)
  line L38 (24, 19.2) -> (27.5, 21.9)
  line L39 (27.5, 21.9) -> (31.000001, 19.2)
  line L40 (38.000001, 3) -> (38.000001, -3)
  line L41 (38.000001, -3) -> (31, -3)
  line L42 (31, -3) -> (31, 3)
  line L43 (31, 3) -> (34.5, 5.7)
  line L44 (34.5, 5.7) -> (38.000001, 3)
  line L45 (10, 24.6) -> (6.5, 21.9)
  line L46 (6.5, 21.9) -> (3, 24.6)
  line L47 (3, 24.6) -> (6.5, 27.3)
  line L48 (6.5, 27.3) -> (10, 24.6)
  line L49 (17, 19.2) -> (13.5, 16.5)
  line L50 (13.5, 16.5) -> (10, 19.2)
  line L51 (10, 19.2) -> (13.5, 21.9)
  line L52 (13.5, 21.9) -> (17, 19.2)
  line L53 (31.000001, 30) -> (27.5, 27.3)
  line L54 (27.5, 27.3) -> (24.000001, 30)
  line L55 (24.000001, 30) -> (31.000001, 30)
  line L56 (34.500001, 21.9) -> (31, 24.6)
  line L57 (31, 24.6) -> (34.5, 27.3)
  line L58 (34.5, 27.3) -> (38.000001, 24.6)
  line L59 (38.000001, 24.6) -> (34.500001, 21.9)
  line L60 (24, 3) -> (24, -3)
  line L61 (24, -3) -> (17, -3)
  line L62 (17, -3) -> (17, 3)
  line L63 (17, 3) -> (20.5, 5.7)
  line L64 (20.5, 5.7) -> (24, 3)
  line L65 (0, 37) -> (0, 30)
  line L66 (0, 30) -> (41.000001, 30)
  line L67 (41.000001, 30) -> (38.000001, 30)
  line L68 (38.000001, 30) -> (38.000001, -3)
  line L69 (38.000001, -3) -> (3, -3)
  line L70 (3, -3) -> (3, 30)
  dimension "d106" = 7
  constraint coincident L2.end L3.start
  constraint coincident L3 L65.end
  constraint perpendicular L1 L66
  constraint perpendicular L67 L68
  constraint coincident L5.end L6.start
  constraint perpendicular L69 L70
  measures "d106" distance of L2.end L65.end
extrude "Extrude21" cut sketch "Sketch12" against normal blind 10 contours L4 L7 L8 L9 L10 L42 L43 L44 L53 L54 L60 L62 L63 L64 L66 L68 L69 L70 picked at (14.666667, -1)
sketch "Sketch13" plane through (0, 21, 0) normal (0, 1, 0) x (-1, 0, 0)
  line L0 (-24.000001, -3) -> (-24.000001, 3)
  line L1 (-24.000001, 3) -> (-20.5, 5.7)
  line L2 (-20.5, 5.7) -> (-17.000001, 3)
  line L3 (-17.000001, 3) -> (-17.000001, -3)
  line L4 (-17.000001, -3) -> (-24.000001, -3)
  line L5 (-10, -3) -> (-10, 3)
  line L6 (-10, 3) -> (-6.5, 5.7)
  line L7 (-6.5, 5.7) -> (-3, 3)
  line L8 (-3, 3) -> (-3, -3)
  line L9 (-3, -3) -> (-10, -3)
  line L10 (-10, 13.8) -> (-6.5, 16.5)
  line L11 (-6.5, 16.5) -> (-3, 13.8)
  line L12 (-3, 13.8) -> (-6.5, 11.1)
  line L13 (-6.5, 11.1) -> (-10, 13.8)
  line L14 (-20.5, 11.1) -> (-24, 13.8)
  line L15 (-24, 13.8) -> (-20.5, 16.5)
  line L16 (-20.5, 16.5) -> (-17, 13.8)
  line L17 (-17, 13.8) -> (-20.5, 11.1)
  line L18 (-27.5, 5.7) -> (-31, 8.4)
  line L19 (-31, 8.4) -> (-27.5, 11.1)
  line L20 (-27.5, 11.1) -> (-24, 8.4)
  line L21 (-24, 8.4) -> (-27.5, 5.7)
  line L22 (-20.500001, 21.9) -> (-24.000001, 24.6)
  line L23 (-24.000001, 24.6) -> (-20.500001, 27.3)
  line L24 (-20.500001, 27.3) -> (-17.000001, 24.6)
  line L25 (-17.000001, 24.6) -> (-20.500001, 21.9)
  line L26 (-31.000001, 3) -> (-31.000001, -3)
  line L27 (-31.000001, -3) -> (-38.000001, -3)
  line L28 (-38.000001, -3) -> (-38.000001, 3)
  line L29 (-38.000001, 3) -> (-34.5, 5.7)
  line L30 (-34.5, 5.7) -> (-31.000001, 3)
  line L31 (-27.500001, 16.5) -> (-31.000001, 19.2)
  line L32 (-31.000001, 19.2) -> (-27.500001, 21.9)
  line L33 (-27.500001, 21.9) -> (-24.000001, 19.2)
  line L34 (-24.000001, 19.2) -> (-27.500001, 16.5)
  line L35 (-13.5, 16.5) -> (-17, 19.2)
  line L36 (-17, 19.2) -> (-13.5, 21.9)
  line L37 (-13.5, 21.9) -> (-10, 19.2)
  line L38 (-10, 19.2) -> (-13.5, 16.5)
  line L39 (-10, 24.6) -> (-6.5, 27.3)
  line L40 (-6.5, 27.3) -> (-3, 24.6)
  line L41 (-3, 24.6) -> (-6.5, 21.9)
  line L42 (-6.5, 21.9) -> (-10, 24.6)
  line L43 (-34.500001, 11.1) -> (-38.000001, 13.8)
  line L44 (-38.000001, 13.8) -> (-34.500001, 16.5)
  line L45 (-34.500001, 16.5) -> (-31.000001, 13.8)
  line L46 (-31.000001, 13.8) -> (-34.500001, 11.1)
  line L47 (-13.5, 5.7) -> (-17, 8.4)
  line L48 (-17, 8.4) -> (-13.5, 11.1)
  line L49 (-13.5, 11.1) -> (-10, 8.4)
  line L50 (-10, 8.4) -> (-13.5, 5.7)
  line L51 (-34.500001, 21.9) -> (-38.000001, 24.6)
  line L52 (-38.000001, 24.6) -> (-34.500001, 27.3)
  line L53 (-34.500001, 27.3) -> (-31.000001, 24.6)
  line L54 (-31.000001, 24.6) -> (-34.500001, 21.9)
  line L55 (-27.500001, 27.3) -> (-31.000001, 30)
  line L56 (-31.000001, 30) -> (-24.000001, 30)
  line L57 (-24.000001, 30) -> (-27.500001, 27.3)
  line L58 (-13.500001, 27.3) -> (-17.000001, 30)
  line L59 (-17.000001, 30) -> (-10.000001, 30)
  line L60 (-10.000001, 30) -> (-13.500001, 27.3)
  line L61 (-41, -5) -> (0, -5)
  line L62 (0, -5) -> (0, 37)
  line L63 (0, 37) -> (-41, 37)
  line L64 (-41, 37) -> (-41, -5)
  line L65 (-41, 37) -> (-41, 30)
  line L66 (-41, 30) -> (0, 30)
  line L67 (0, 30) -> (-3, 30)
  line L68 (-3, 30) -> (-3, -3)
  line L69 (-3, -3) -> (-38.000001, -3)
  line L70 (-38.000001, -3) -> (-38.000001, 30)
  dimension "d109" = 7
  constraint coincident L63.end L64.start
  constraint perpendicular L63 L65
  constraint coincident L62 L66.end
  constraint perpendicular L62 L66
  constraint coincident L66 L67.end
  constraint coincident L8.end L9.start
  constraint perpendicular L9 L68
  constraint perpendicular L66 L70
  measures "d109" distance of L63.end L65.end
extrude "Extrude22" cut sketch "Sketch13" against normal blind 10 contours L0 L1 L2 L3 L5 L6 L7 L26 L29 L30 L55 L57 L58 L60 L66 L68 L69 L70 picked at (-14.666667, 1)
extrude "Extrude23" add 2 faces at (3, 1, 8) (3, 20, 12.333333) along direction (1, 0, 0) blind 13
sketch "Sketch14" plane through (16, 0, 0) normal (1, 0, 0) x (0, 1, 0)
  line L0 (0, -3) -> (3, -3)
  line L1 (3, -3) -> (3, 30)
  line L2 (3, 30) -> (0, 30)
  line L3 (0, 30) -> (0, -3)
sketch "Sketch15" plane through (0, 0, 0) normal (0, -1, 0) x (1, 0, 0)
  line L0 (0, -5) -> (41, -5)
  line L1 (41, -5) -> (41, 37)
  line L2 (41, 37) -> (0, 37)
  line L3 (0, 37) -> (0, -5)
  line L4 (38.000001, -3) -> (16, -3)
  line L5 (16, -3) -> (16, 30)
  line L6 (16, 30) -> (38.000001, 30)
  line L7 (38.000001, 30) -> (38.000001, -3)
  line L8 (38.000001, 30) -> (41.000001, 30)
  line L9 (38.000001, -3) -> (41.000001, -3)
  constraint perpendicular L1 L8
  constraint perpendicular L1 L9
extrude "Extrude24" cut sketch "Sketch15" against normal blind 10 contours L1 L7 L8 L9 picked at (39, 19)
sketch "Sketch16" plane through (0, 21, 0) normal (0, 1, 0) x (-1, 0, 0)
  line L0 (-16, -3) -> (-38.000001, -3)
  line L1 (-38.000001, -3) -> (-38.000001, 30)
  line L2 (-38.000001, 30) -> (-16, 30)
  line L3 (-16, 30) -> (-16, -3)
  line L4 (-41, -5) -> (0, -5)
  line L5 (0, -5) -> (0, 37)
  line L6 (0, 37) -> (-41, 37)
  line L7 (-41, 37) -> (-41, -5)
  line L8 (-41.000001, 30) -> (-38.000001, 30)
  line L9 (-38.000001, -3) -> (-41.000001, -3)
  constraint perpendicular L1 L8
  constraint perpendicular L1 L9
extrude "Extrude25" cut sketch "Sketch16" against normal blind 10 contours L1 L7 L8 L9 picked at (-39, 8)
extrude "Extrude26" cut sketch "Sketch14" 1 faces at (16, 20, 12.333333) against normal blind 5 contours L0 L1 L2 L3 picked at (1, 8)
extrude "Extrude27" add 1 faces at (19.333333, 20, -5) along direction (0, 0, -1) blind 1
sketch "Sketch17" plane through (0, 0, 37) normal (0, 0, 1) x (-1, 0, 0)
  line L0 (-37, -6) -> (-15, -8.5)
  arc A0 (-15, -12.5) -> (-15, -8.5) centre (-15, -10.5) ccw
  line L1 (-15, -12.5) -> (-37, -15)
  line L2 (-37, -15) -> (-37, -6)
  line L3 (0, -21) -> (0, 0)
  line L4 (0, 0) -> (-41, 0)
  line L5 (-41, 0) -> (-41, -21)
  line L6 (-41, -21) -> (0, -21)
  line L7 (-41, -21) -> (-41, -10.5)
  line L8 (-41, -10.5) -> (-34.000001, -10.5)
  circle A1 centre (-34.000001, -10.5) radius 10.5
  dimension "d122" = 21
  constraint coincident L5.end L6.start
  constraint midpoint L5 L7.end
  constraint perpendicular L2 L8
  measures "d122" diameter of A1
extrude "Extrude28" cut sketch "Sketch17" against normal blind 10 contours L4 L5 A1 | L5 L6 L7 A1 picked at (-40.595809, -1.47091) picked at (-40.595809, -19.52909)
extrude "Extrude29" add 1 faces at (4.666667, 3, 19) along direction (0, 1, 0) blind 1
extrude "Extrude30" add 4 faces at (1, 18, 12.333333) (8, 18, 16.666667) (5.666667, 18, 1) (5.666667, 18, 5.333333) along direction (0, -1, 0) blind 1
extrude "Extrude31" cut 4 faces at (1, 17, 12.333333) (8, 17, 16.666667) (6.444445, 17, 1) (5.666667, 17, 5.333333) along direction (0, 1, 0) blind 2
extrude "Extrude32" cut 1 faces at (5.444444, 4, 19) along direction (0, -1, 0) blind 2
extrude "Extrude33" add 1 faces at (3.666667, 21, 20.333333) along direction (0, 1, 0) blind 2
extrude "Extrude34" add 1 faces at (3.666667, 0, 20.333333) along direction (0, -1, 0) blind 2
sketch "Sketch18" plane through (0, 0, 37) normal (0, 0, 1) x (-1, 0, 0)
  line L0 (-37, -6) -> (-15, -8.5)
  arc A0 (-15, -12.5) -> (-15, -8.5) centre (-15, -10.5) ccw
  line L1 (-15, -12.5) -> (-37, -15)
  line L2 (-37, -15) -> (-37, -6)
  arc A1 (-41, -18.326238) -> (-34.000001, -21) centre (-34.000001, -10.5) ccw
  line L3 (-34.000001, -21) -> (-34.000001, -23)
  line L4 (-34.000001, -23) -> (0, -23)
  line L5 (0, -23) -> (0, 2)
  line L6 (0, 2) -> (-34.000001, 2)
  line L7 (-34.000001, 2) -> (-34.000001, 0)
  arc A2 (-34.000001, 0) -> (-41, -2.673762) centre (-34.000001, -10.5) ccw
  line L8 (-41, -2.673762) -> (-41, -18.326238)
  line L9 (-34.000001, 2) -> (-41.000001, 2)
  line L10 (-41.000001, 2) -> (-41, -2.673762)
  constraint perpendicular L7 L9
extrude "Extrude35" add sketch "Sketch18" against normal blind 7 contours L7 A2 L9 L10 picked at (-37.340507, 1.185288)
sketch "Sketch19" plane through (0, 0, 37) normal (0, 0, 1) x (-1, 0, 0)
  line L0 (-37, -6) -> (-15, -8.5)
  arc A0 (-15, -12.5) -> (-15, -8.5) centre (-15, -10.5) ccw
  line L1 (-15, -12.5) -> (-37, -15)
  line L2 (-37, -15) -> (-37, -6)
  arc A1 (-41, -18.326238) -> (-34.000001, -21) centre (-34.000001, -10.5) ccw
  line L3 (-34.000001, -21) -> (-34.000001, -23)
  line L4 (-34.000001, -23) -> (0, -23)
  line L5 (0, -23) -> (0, 2)
  line L6 (0, 2) -> (-41.000001, 2)
  line L7 (-41.000001, 2) -> (-41, -2.673762)
  line L8 (-41, -2.673762) -> (-41, -18.326238)
  line L9 (-34.000001, -23) -> (-41.000001, -23)
  line L10 (-41.000001, -23) -> (-41, -18.326238)
  constraint perpendicular L3 L9
extrude "Extrude36" add sketch "Sketch19" against normal blind 7 contours A1 L3 L9 L10 picked at (-37.340507, -22.185288)
fillet "Fillet1" radius 5 2 edges at (41.000001, -2, 33.5) (41.000001, 23, 33.5)
fillet "Fillet2" radius 2 2 edges at (5.5, 2, 30) (5.5, 19, 30)
sketch "Sketch20" plane through (0, 0, -3) normal (0, 0, 1) x (-1, 0, 0)
  line L0 (-3, -3) -> (-3, -6)
  line L1 (-3, -6) -> (-6.5, -4.5)
  line L2 (-6.5, -4.5) -> (-3, -3)
  line L3 (0, -19) -> (0, -2)
  line L4 (0, -2) -> (-11, -2)
  line L5 (-11, -2) -> (-11, 2)
  line L6 (-11, 2) -> (-41.000001, 2)
  line L7 (-41.000001, 2) -> (-41.000001, -23)
  line L8 (-41.000001, -23) -> (-11, -23)
  line L9 (-11, -23) -> (-11, -19)
  line L10 (-11, -19) -> (0, -19)
  line L11 (-3, -15) -> (-3, -18)
  line L12 (-3, -18) -> (-6.5, -16.5)
  line L13 (-6.5, -16.5) -> (-3, -15)
  line L14 (-38, -12) -> (-34.5, -13.5)
  line L15 (-34.5, -13.5) -> (-38, -15)
  line L16 (-38, -15) -> (-38, -12)
  line L17 (-17.000001, -18) -> (-20.5, -16.5)
  line L18 (-20.5, -16.5) -> (-17, -15)
  line L19 (-17, -15) -> (-13.5, -16.5)
  line L20 (-13.5, -16.5) -> (-17.000001, -18)
  line L21 (-24, -12) -> (-20.5, -13.5)
  line L22 (-20.5, -13.5) -> (-24, -15)
  line L23 (-24, -15) -> (-27.5, -13.5)
  line L24 (-27.5, -13.5) -> (-24, -12)
  line L25 (-27.5, -10.5) -> (-31, -12)
  line L26 (-31, -12) -> (-34.5, -10.5)
  line L27 (-34.5, -10.5) -> (-31, -9)
  line L28 (-31, -9) -> (-27.5, -10.5)
  line L29 (-17, -12) -> (-20.5, -10.5)
  line L30 (-20.5, -10.5) -> (-17, -9)
  line L31 (-17, -9) -> (-13.5, -10.5)
  line L32 (-13.5, -10.5) -> (-17, -12)
  line L33 (-10, -12) -> (-6.5, -13.5)
  line L34 (-6.5, -13.5) -> (-10, -15)
  line L35 (-10, -15) -> (-13.5, -13.5)
  line L36 (-13.5, -13.5) -> (-10, -12)
  line L37 (-31.000001, -18) -> (-34.5, -16.5)
  line L38 (-34.5, -16.5) -> (-31, -15)
  line L39 (-31, -15) -> (-27.5, -16.5)
  line L40 (-27.5, -16.5) -> (-31.000001, -18)
  line L41 (-3, -12) -> (-6.5, -10.5)
  line L42 (-6.5, -10.5) -> (-3, -9)
  line L43 (-3, -9) -> (-3, -12)
  line L44 (-10, -9) -> (-13.5, -7.5)
  line L45 (-13.5, -7.5) -> (-10, -6)
  line L46 (-10, -6) -> (-6.5, -7.5)
  line L47 (-6.5, -7.5) -> (-10, -9)
  line L48 (-24, -9) -> (-27.5, -7.5)
  line L49 (-27.5, -7.5) -> (-24, -6)
  line L50 (-24, -6) -> (-20.5, -7.5)
  line L51 (-20.5, -7.5) -> (-24, -9)
  line L52 (-17, -3) -> (-13.5, -4.5)
  line L53 (-13.5, -4.5) -> (-17, -6)
  line L54 (-17, -6) -> (-20.5, -4.5)
  line L55 (-20.5, -4.5) -> (-17, -3)
  line L56 (-31, -3) -> (-27.5, -4.5)
  line L57 (-27.5, -4.5) -> (-31, -6)
  line L58 (-31, -6) -> (-34.5, -4.5)
  line L59 (-34.5, -4.5) -> (-31, -3)
  line L60 (-38, -6) -> (-34.5, -7.5)
  line L61 (-34.5, -7.5) -> (-38, -9)
  line L62 (-38, -9) -> (-38, -6)
  line L63 (-3, -18) -> (-6.5, -16.5)
  line L64 (-3, -15) -> (-6.5, -16.5)
  line L65 (-3, -15) -> (-3, -18)
  line L66 (-3, -12) -> (-6.5, -10.5)
  line L67 (-6.5, -10.5) -> (-3, -9)
  line L68 (-3, -9) -> (-3, -12)
  line L69 (-3, -6) -> (-6.5, -4.5)
  line L70 (-6.5, -4.5) -> (-3, -3)
  line L71 (-3, -3) -> (-3, -6)
  constraint coincident L11.end L12.start
  constraint coincident L12.end L13.start
  constraint coincident L11.start L13.end
  constraint coincident L41.start L43.end
  constraint coincident L41.end L42.start
  constraint coincident L42.end L43.start
  constraint coincident L0.end L1.start
  constraint coincident L1.end L2.start
  constraint coincident L0.start L2.end
extrude "Extrude37" add sketch "Sketch20" against normal blind 3 contours L0 L1 L2 L69 L70 L71 | L11 L12 L13 L63 L64 L65 | L41 L42 L43 L66 L67 L68 picked at (-4.166667, -4.5) picked at (-4.166667, -16.5) picked at (-4.166667, -10.5)
fillet "Fillet3" radius 2 2 edges at (5.5, 2, -3) (5.5, 19, -3)
fillet "Fillet4" radius 2 2 edges at (11, 20, -3) (11, 1, -3)
fillet "Fillet5" radius 2 2 edges at (11, 1, 30) (11, 20, 30)
equation "d49 = 1.5 mm + 4 mm"
